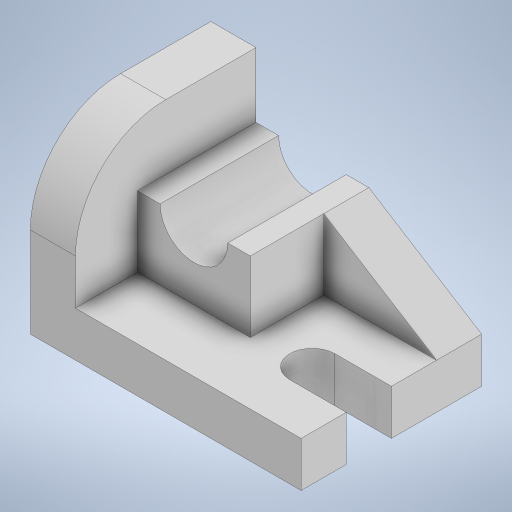
# Autodesk Inventor part: desenho 1
Saved by Autodesk Inventor 2024 (Build 280153000, 153)
## iProperties
Created: 2023-09-18
Part Number: desenho 1
Material: Generic
Document SubType Name: Modeling
Designer: LORAC
Density: 1 g/cm^3
Appearance: Default
Author: LORAC
Autodesk Inventor part; units mm, degrees
ref_plane "YZ Plane" through (0, 0, 0) normal (1, 0, 0) x (0, 1, 0)
ref_plane "XZ Plane" through (0, 0, 0) normal (0, 1, 0) x (-1, 0, 0)
ref_plane "XY Plane" through (0, 0, 0) normal (0, 0, 1) x (1, 0, 0)
sketch "Sketch1" plane through (0, 0, 0) normal (0, 1, 0) x (-1, 0, 0)
  line L0 (-48, 32) -> (48, 32)
  line L1 (48, 32) -> (48, -32)
  line L2 (48, -32) -> (-48, -32)
  line L3 (-48, -32) -> (-48, 32)
  line L4 (-48, 32) -> (48, -32) construction
  line L5 (48, 32) -> (-48, -32) construction
  line L6 (-48, 16) -> (-28, 16)
  line L7 (-28, 0) -> (-48, 0)
  arc A0 (-28, 0) -> (-28, 16) centre (-28, 8) ccw
  point P0 (0, 0)
  point P1 (-38, 0)
  dimension "d0" = 96
  dimension "d1" = 64
  dimension "d3" = 16
  dimension "d4" = 16
  constraints: 16 end point, 4 midpoint, 2 horizontal, 2 parallel, 2 point on circle, 1 centre point, 1 perpendicular, 1 point on line
  measures "d0" distance of L1.end L2.end
  measures "d1" distance of L0.end L1.end
  measures "d3" distance between parallel lines of L0 L6
  measures "d4" distance from line of point (-38, 0) L6
extrude "Extrusion1" add sketch "Sketch1" along normal blind 16 contours L0 L1 L2 L3 L7 A0 L6
sketch "Sketch2" plane through (0, 16, 0) normal (0, 1, 0) x (1, 0, 0)
  line L0 (-48, 32) -> (-48, -32) projected
  line L1 (-48, -32) -> (48, -32) projected
  line L2 (-48, 32) -> (-32, 32)
  line L3 (-32, 32) -> (-32, -32)
  line L4 (-32, -32) -> (-48, -32)
  line L5 (-48, -32) -> (-48, 32)
  point P0 (0, 0)
  dimension "d8" = 16
  constraints: 8 end point, 2 parallel, 1 horizontal, 1 perpendicular, 1 point on line
  measures "d8" distance of L3.end L4.end
extrude "Extrusion2" add sketch "Sketch2" along normal blind 48
fillet "Fillet1" radius 32 1 edges at (-40, 64, 32)
sketch "Sketch3" plane through (48, 0, -32) normal (0, 0, -1) x (-1, 0, 0)
  line L0 (80, 16) -> (0, 16) projected
  line L1 (80, 16) -> (40, 16)
  line L2 (40, 16) -> (40, 41)
  line L3 (80, 41) -> (80, 16)
  arc A0 (48, 41) -> (72, 41) centre (60, 41) ccw
  line L4 (40, 41) -> (48, 41)
  line L5 (72, 41) -> (80, 41)
  point P0 (48, 0)
  dimension "d12" = 40
  dimension "d13" = 25
  constraints: 10 end point, 3 parallel, 2 point on circle, 1 centre point, 1 horizontal, 1 perpendicular
  measures "d12" distance of L2.end L3.start
  measures "d13" distance of L1.end L2.end
extrude "Extrusion3" add sketch "Sketch3" against normal blind 42
sketch "Sketch4" plane through (48, 0, -32) normal (0, 0, -1) x (-1, 0, 0)
  line L0 (80, 16) -> (0, 16) projected
  line L1 (40, 41) -> (48, 41) projected
  line L2 (0, 16) -> (40, 41)
  line L3 (40, 16) -> (80, 16) projected
  line L4 (40, 41) -> (40, 16)
  line L5 (40, 16) -> (0, 16)
  point P0 (48, 0)
  constraints: 6 end point, 2 perpendicular
extrude "Extrusion4" add sketch "Sketch4" against normal blind 16
body "Solid1"
